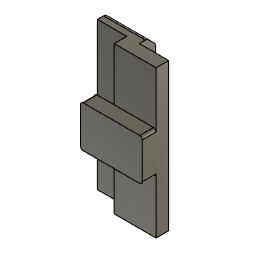
detent tab modification (Autodesk Fusion 360 design; units mm, degrees)
Autodesk Fusion 360 part; units mm, degrees
sketch "Sketch1" plane through (0, 0, 0) normal (0, 1, 0) x (1, 0, 0)
  line L0 (3.68, -2.475) -> (-3.68, -2.475)
  line L1 (-3.68, -2.475) -> (-3.68, 2.475)
  line L2 (-3.68, 2.475) -> (3.68, 2.475)
  line L3 (3.68, 2.475) -> (3.68, -2.475)
  line L4 (3.68, -2.475) -> (-3.68, 2.475) construction
  line L5 (-3.68, -2.475) -> (3.68, 2.475) construction
  dimension "d124" = 7.36
  dimension "d125" = 4.95
  constraint horizontal L0
  constraint perpendicular L0 L1
  constraint parallel L0 L2
  constraint parallel L1 L3
  constraint coincident L4 origin
  constraint coincident L5 origin
  measures "d124" distance of L0.start L0.end
  measures "d125" distance of L0.start L2.end
extrude "Extrude1" add sketch "Sketch1" along normal blind 1.65 makes body 1
fillet "Fillet1" radius 0.3 4 edges at (-3.68, 0.825, 2.475) (3.68, 0.825, 2.475) (3.68, 0.825, -2.475) (-3.68, 0.825, -2.475) on bodies 1
sketch "Sketch2" plane through (0, 1.65, 0) normal (0, 1, 0) x (-1, 0, 0)
  line L0 (1.32, 8.795) -> (-3.68, 8.795)
  line L1 (-3.68, 8.795) -> (-3.68, -8.795)
  line L2 (-3.68, -8.795) -> (1.32, -8.795)
  line L3 (1.32, -8.795) -> (1.32, 8.795)
  line L4 (-3.68, 2.175) -> (-3.68, -2.175)
  line L5 (0, 0) -> (-3.68, 0) construction
  dimension "d136" = 17.59
  dimension "d137" = 5
  constraint horizontal L0
  constraint vertical L1
  constraint horizontal L2
  constraint vertical L3
  constraint collinear L1 L4
  constraint coincident L5.start origin
  constraint perpendicular L4 L5
  constraint coincident L1 L5.end
  constraint symmetric L0 L2 L5
  measures "d136" distance of L0 L2
  measures "d137" distance of L1.end L2.end
extrude "Extrude5" add sketch "Sketch2" along normal blind 1.5 bodies 1
sketch "Sketch6" plane through (0, 3.15, 0) normal (0, 1, 0) x (-1, 0, 0)
  line L0 (-3.68, 8.795) -> (-3.68, -8.795)
  line L1 (-3.68, -8.795) -> (1.32, -8.795)
  line L2 (1.32, -8.795) -> (1.32, 8.795)
  line L3 (1.32, 8.795) -> (-3.68, 8.795)
  line L4 (-0.18, 8.795) -> (4.82, 8.795)
  line L5 (4.82, 8.795) -> (4.82, -8.795)
  line L6 (4.82, -8.795) -> (-0.18, -8.795)
  line L7 (-0.18, -8.795) -> (-0.18, 8.795)
  dimension "d158" = 3.5
  constraint horizontal L4
  constraint vertical L5
  constraint horizontal L6
  constraint vertical L7
  constraint collinear L1 L6
  constraint collinear L3 L4
  constraint equal L1 L6
  measures "d158" distance of L2 L5
extrude "Extrude7" add sketch "Sketch6" along normal blind 1.95 separate body contours L1 L2 L3 L4 L6 L7 | L2 L4 L5 L6 makes body 2
chamfer "Chamfer2" distance 1 angle 45 2 edges at (-2.32, 5.1, 8.795) (-2.32, 5.1, -8.795) on bodies 2
fillet "Fillet3" radius 0.5 4 edges at (-2.32, 5.1, 7.795) (-2.32, 4.1, 8.795) (-2.32, 5.1, -7.795) (-2.32, 4.1, -8.795) on bodies 2
combine "Combine1" operation add target body 2 tool bodies 1
sketch "Sketch7" plane through (0, 0, 0) normal (0, -1, 0) x (1, 0, 0)
  arc A0 (-3.68, -2.175) -> (-3.38, -2.475) centre (-3.38, -2.175) ccw
  line L0 (-3.38, -2.475) -> (3.38, -2.475)
  arc A1 (3.38, -2.475) -> (3.68, -2.175) centre (3.38, -2.175) ccw
  line L1 (3.68, -2.175) -> (3.68, 2.175)
  arc A2 (3.68, 2.175) -> (3.38, 2.475) centre (3.38, 2.175) ccw
  line L2 (3.38, 2.475) -> (-3.38, 2.475)
  arc A3 (-3.38, 2.475) -> (-3.68, 2.175) centre (-3.38, 2.175) ccw
  line L3 (-3.68, 2.175) -> (-3.68, -2.175)
extrude "Extrude8" [suppressed]
equation "d131 = DetentBottomPieceFilletRadius"
equation "d158 = DetentShiftDistance"
equation "DetentBottomPieceFilletRadius = 0.3 mm"
equation "DetentShiftDistance = 3.5 mm"
